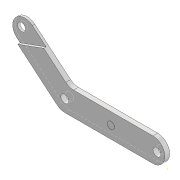
# Autodesk Inventor part: GripP1
Saved by Autodesk Inventor 2021 (Build 250183000, 183)
## iProperties
Created: 2022-09-30
Part Number: GripP1
Material: Generic
Document SubType Name: Modeling
Designer: brian
Density: 1 g/cm^3
Appearance: Default
Mass: 33.1463 g
Surface Area: 148.126 cm^2
Volume: 33.1463 cm^3
d0: 30,000 mm
d2: 30,000 mm
d3: 50,00 deg
d4: 120,000 mm
d5: 90,000 mm
d6: 10,000 mm
d7: 10,000 mm
d8: 10,000 mm
d9: 10,000 mm
d10: 15,000 mm
d11: 3,000 mm
d12: 0,00 deg
d13: 10,000 mm
Author: brian
Autodesk Inventor part; units mm, degrees
ref_plane "YZ Plane" through (0, 0, 0) normal (1, 0, 0) x (0, 1, 0)
ref_plane "XZ Plane" through (0, 0, 0) normal (0, 1, 0) x (-1, 0, 0)
ref_plane "XY Plane" through (0, 0, 0) normal (0, 0, 1) x (1, 0, 0)
sketch "Sketch1" plane through (0, 0, 0) normal (0, 0, 1) x (1, 0, 0)
  line L0 (-15, 0) -> (-125.4596, 0)
  line L1 (-130.9191, 0) -> (-130.9191, 30)
  line L2 (-114.5404, 30) -> (-15, 30)
  line L3 (0, 15) -> (0, 15)
  line L4 (-130.9191, 0) -> (-111.6355, 22.9813)
  line L5 (-111.6355, 22.9813) -> (-120, 30)
  line L6 (-190.2213, 69.3416) -> (-190.2213, 69.3416)
  line L7 (-188.3724, 48.2091) -> (-135.1014, 3.5093)
  line L8 (-124.1823, 33.5093) -> (-169.0888, 71.1904)
  circle A0 centre (-182.5608, 62.9137) radius 5
  circle A1 centre (-10, 15) radius 5
  arc A2 (0, 15) -> (-15, 30) centre (-15, 15) ccw
  arc A3 (-15, 0) -> (0, 15) centre (-15, 15) ccw
  arc A4 (-169.0888, 71.1904) -> (-190.2213, 69.3416) centre (-178.7306, 59.6997) ccw
  arc A5 (-190.2213, 69.3416) -> (-188.3724, 48.2091) centre (-178.7306, 59.6997) ccw
  arc A6 (-124.1823, 33.5093) -> (-114.5404, 30) centre (-114.5404, 45) ccw
  arc A7 (-135.1014, 3.5093) -> (-125.4596, 0) centre (-125.4596, 15) ccw
  line L9 (-15, 15) -> (-82.4661, 15) construction
  line L10 (-178.7306, 59.6997) -> (-70.1019, -31.4506) construction
  circle A8 centre (-125.4596, 15) radius 5
  point P0 (0, 0)
  point P1 (0, 30)
  point P2 (-199.8631, 57.8509)
  point P3 (0, 15)
  point P4 (-190.2213, 69.3416)
  dimension "d0" = 30
  dimension "d2" = 30
  dimension "d3" = 50
  dimension "d4" = 120
  dimension "d5" = 90
  dimension "d6" = 10
  dimension "d7" = 10
  dimension "d8" = 10
  dimension "d9" = 10
  dimension "d10" = 15
  dimension "d13" = 10
  dimension "d14" = 15
  dimension "d15" = 15
  constraints: 22 end point, 12 point on circle, 12 tangent, 11 point on line, 9 centre point, 6 parallel, 5 equal radius, 3 perpendicular, 2 horizontal, 1 coincident
  measures "d0" distance of point (0, 30) point (0, 0)
  measures "d2" distance of L1.start L4.end
  measures "d3" angle of L0 L4
  measures "d4" distance of L5.end point (0, 30)
  measures "d5" distance of point (-199.863, 57.851) L1.start
  measures "d6" diameter of A0
  measures "d7" distance from line of L6 A0.centre
  measures "d8" diameter of A1
  measures "d9" distance from line of L3 A1.centre
  measures "d10" radius of A2
  measures "d13" diameter of A8
  measures "d14" distance from line of L2 A1.centre
  measures "d15" distance from line of L8 A0.centre
extrude "Extrusion1" add sketch "Sketch1" along normal blind 3 contours L0 A7 L7 A5 A4 L8 A6 L2 A2 A3
sketch "Sketch2" plane through (0, 0, 3) normal (0, 0, 1) x (1, 0, 0)
  point P0 (0, 0)
sketch "Sketch3" plane through (0, 0, 3) normal (0, 0, 1) x (1, 0, 0)
  line L0 (-125.4596, 0) -> (-15, 0) projected
  arc A0 (-15, 0) -> (-15, 30) centre (-15, 15) ccw projected
  line L1 (-15, 30) -> (-114.5404, 30) projected
  arc A1 (-124.1823, 33.5093) -> (-114.5404, 30) centre (-114.5404, 45) ccw projected
  line L2 (-124.1823, 33.5093) -> (-169.0888, 71.1904) projected
  arc A2 (-169.0888, 71.1904) -> (-188.3724, 48.2091) centre (-178.7306, 59.6997) ccw projected
  line L3 (-188.3724, 48.2091) -> (-135.1014, 3.5093) projected
  arc A3 (-135.1014, 3.5093) -> (-125.4596, 0) centre (-125.4596, 15) ccw projected
  circle A4 centre (-125.4596, 15) radius 5 projected
  circle A5 centre (-10, 15) radius 5 projected
  circle A6 centre (-182.5608, 62.9137) radius 5 projected
  line L4 (-248.5616, 21.4167) -> (-81.5166, 82.2161)
  line L5 (-124.1823, 33.5093) -> (-169.0888, 71.1904) projected
  point P0 (0, 0)
  point P1 (-151.7599, 56.6497)
  point P2 (-151.7599, 56.6497)
  point P3 (-184.3118, 44.8018)
  dimension "d16" = 60
  dimension "d17" = 36
  constraints: 2 end point, 2 point on line
  measures "d16" angle of L4 L2
  measures "d17" distance of L2.start point (-151.76, 56.65)
extrude "Extrusion2" add sketch "Sketch3" along normal blind 3 contours A3 L3 L4 L2 A1 L1 A0 L0
sketch "Sketch4" plane through (0, 0, 0) normal (0, 0, -1) x (-1, 0, 0)
  circle A0 centre (182.5608, 62.9137) radius 5 projected
  point P0 (0, 0)
extrude "Extrusion3" [suppressed]
sketch "Sketch5" plane through (0, 0, 6) normal (0, 0, 1) x (1, 0, 0)
  circle A0 centre (-67.7298, 15) radius 2.5
  circle A1 centre (-10, 15) radius 5 projected
  circle A2 centre (-125.4596, 15) radius 5 projected
  point P0 (0, 0)
  dimension "d22" = 115.4595
  dimension "d23" = 57.7298
  dimension "d28" = 5
  constraints: 1 centre point, 1 horizontal alignment
  measures "d22" distance of A2.centre A1.centre
  measures "d23" distance of A0.centre A2.centre
  measures "d28" diameter of A0
extrude "Extrusion4" cut sketch "Sketch5" against normal blind 0.1 contours A0
sketch "Sketch6" plane through (0, 0, 0) normal (0, 0, -1) x (-1, 0, 0)
  circle A0 centre (67.7298, 15) radius 2.5 projected
  point P0 (0, 0)
extrude "Extrusion5" cut sketch "Sketch6" against normal blind 0.1
equation "\"d2\" = d0"
equation "\"d7\" = d6"
equation "\"d8\" = d6"
equation "\"d9\" = d7"
equation "\"d10\" = 0.5 * d0"
equation "\"d13\" = d8"
equation "\"d14\" = 0.5 * d0"
equation "\"d15\" = d14"
equation "\"d17\" = 1.2 * d0"
equation "\"d18\" = d11"
equation "\"d20\" = 4 * d11"
equation "\"d23\" = 0.5 * d22"
equation "\"d11\" = 3"
body "Solid1"
